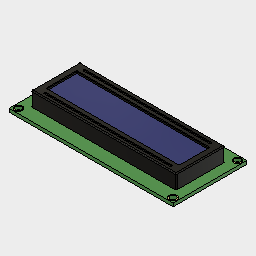
lcd_16x2 (Autodesk Fusion 360 design; units mm, degrees)
Autodesk Fusion 360 part; units mm, degrees
sketch "Sketch1" plane through (0, 0, 0) normal (0, 1, 0) x (1, 0, 0)
  line L0 (40, -18) -> (-40, -18)
  line L1 (-40, -18) -> (-40, 18)
  line L2 (-40, 18) -> (40, 18)
  line L3 (40, 18) -> (40, -18)
  line L4 (-40, -18) -> (40, 18) construction
  circle A0 centre (-37.7, 15.7) radius 1.4
  circle A1 centre (-37.7, -15.7) radius 1.4
  circle A2 centre (37.7, -15.7) radius 1.4
  circle A3 centre (37.7, 15.7) radius 1.4
  circle A4 centre (-32, 15.5) radius 0.5
  circle A5 centre (-29.46, 15.5) radius 0.5
  circle A6 centre (-26.92, 15.5) radius 0.5
  circle A7 centre (-24.38, 15.5) radius 0.5
  circle A8 centre (-21.84, 15.5) radius 0.5
  circle A9 centre (-19.3, 15.5) radius 0.5
  circle A10 centre (-16.76, 15.5) radius 0.5
  circle A11 centre (-14.22, 15.5) radius 0.5
  circle A12 centre (-11.68, 15.5) radius 0.5
  circle A13 centre (-9.14, 15.5) radius 0.5
  circle A14 centre (-6.6, 15.5) radius 0.5
  circle A15 centre (-4.06, 15.5) radius 0.5
  circle A16 centre (-1.52, 15.5) radius 0.5
  circle A17 centre (1.02, 15.5) radius 0.5
  circle A18 centre (3.56, 15.5) radius 0.5
  circle A19 centre (6.1, 15.5) radius 0.5
  dimension "d1" = 80
  dimension "d2" = 36
  dimension "d5" = 2.8
  dimension "d6" = 2.8
  dimension "d7" = 2.8
  dimension "d8" = 2.8
  dimension "d9" = 31.4
  dimension "d10" = 75.4
  dimension "d13" = 1
  dimension "d14" = 8
  dimension "d15" = 2.5
  dimension "d18" = 2.54
  dimension "d19" = 0
  measures "d1" distance of L1.end L2.end
  measures "d2" distance of L0.end L1.end
  measures "d5" diameter of A0
  measures "d6" diameter of A1
  measures "d7" diameter of A2
  measures "d8" diameter of A3
  measures "d9" distance of A0.centre A1.centre
  measures "d10" distance of A1.centre A2.centre
  measures "d13" diameter of A4
  measures "d14" distance of L1 A4.centre
  measures "d15" distance of L2 A4.centre
extrude "Extrude1" add sketch "Sketch1" along normal blind 1.6 makes body 1
sketch "Sketch2" plane through (0, 1.6, 0) normal (0, 1, 0) x (-1, 0, 0)
  circle A0 centre (-3.56, -15.5) radius 0.5
  circle A1 centre (-1.02, -15.5) radius 0.5
  circle A2 centre (1.52, -15.5) radius 0.5
  circle A3 centre (4.06, -15.5) radius 0.5
  circle A4 centre (6.6, -15.5) radius 0.5
  circle A5 centre (-6.1, -15.5) radius 0.5
  circle A6 centre (11.68, -15.5) radius 0.5
  circle A7 centre (24.38, -15.5) radius 0.5
  circle A8 centre (21.84, -15.5) radius 0.5
  circle A9 centre (19.3, -15.5) radius 0.5
  circle A10 centre (16.76, -15.5) radius 0.5
  circle A11 centre (14.22, -15.5) radius 0.5
  circle A12 centre (9.14, -15.5) radius 0.5
  circle A13 centre (26.92, -15.5) radius 0.5
  circle A14 centre (29.46, -15.5) radius 0.5
  circle A15 centre (32, -15.5) radius 0.5
  circle A16 centre (-37.7, -15.7) radius 1.4
  circle A17 centre (-37.7, 15.7) radius 1.4
  circle A18 centre (37.7, 15.7) radius 1.4
  circle A19 centre (37.7, -15.7) radius 1.4
  line L0 (-40, -18) -> (40, -18)
  line L1 (40, -18) -> (40, 18)
  line L2 (40, 18) -> (-40, 18)
  line L3 (-40, 18) -> (-40, -18)
  line L4 (-35.35, 11.9) -> (35.35, 11.9)
  line L5 (35.35, 11.9) -> (35.35, -11.9)
  line L6 (35.35, -11.9) -> (-35.35, -11.9)
  line L7 (-35.35, -11.9) -> (-35.35, 11.9)
  line L8 (-35.35, 11.9) -> (35.35, -11.9) construction
  line L9 (35.35, 11.9) -> (-35.35, -11.9) construction
  line L10 (-32.25, 7.25) -> (32.25, 7.25)
  line L11 (32.25, 7.25) -> (32.25, -7.25)
  line L12 (32.25, -7.25) -> (-32.25, -7.25)
  line L13 (-32.25, -7.25) -> (-32.25, 7.25)
  line L14 (-32.25, 7.25) -> (32.25, -7.25) construction
  line L15 (32.25, 7.25) -> (-32.25, -7.25) construction
  dimension "d20" = 70.7
  dimension "d21" = 23.8
  dimension "d22" = 64.5
  dimension "d23" = 14.5
  measures "d20" distance of L5.end L6.end
  measures "d21" distance of L4.end L5.end
  measures "d22" distance of L11.end L12.end
  measures "d23" distance of L10.end L11.end
extrude "Extrude2" add sketch "Sketch2" along normal blind 6 separate body contours L10 L11 L12 L13 makes body 2
extrude "Extrude3" add sketch "Sketch2" along normal blind 7 separate body contours L4 L5 L6 L7 makes body 3
sketch "Sketch3" plane through (0, 8.6, 0) normal (0, 1, 0) x (-1, 0, 0)
  line L0 (32.25, -7.25) -> (-32.25, -7.25)
  line L1 (-32.25, -7.25) -> (-32.25, 7.25)
  line L2 (-32.25, 7.25) -> (32.25, 7.25)
  line L3 (32.25, 7.25) -> (32.25, -7.25)
  line L4 (-35.35, -11.9) -> (35.35, -11.9)
  line L5 (35.35, -11.9) -> (35.35, 11.9)
  line L6 (35.35, 11.9) -> (-35.35, 11.9)
  line L7 (-35.35, 11.9) -> (-35.35, -11.9)
  line L8 (30.5703, -8.9649) -> (-30.5703, -8.9649)
  arc A0 (-30.5703, -8.9649) -> (-30.5703, -9.9649) centre (-30.5703, -9.4649) ccw
  line L9 (-30.5703, -9.9649) -> (30.5703, -9.9649)
  arc A1 (30.5703, -9.9649) -> (30.5703, -8.9649) centre (30.5703, -9.4649) ccw
  line L10 (30.5703, -9.4649) -> (-30.5703, -9.4649) construction
  line L11 (30.5703, 10.268) -> (-30.5703, 10.268)
  arc A2 (-30.5703, 10.268) -> (-30.5703, 9.268) centre (-30.5703, 9.768) ccw
  line L12 (-30.5703, 9.268) -> (30.5703, 9.268)
  arc A3 (30.5703, 9.268) -> (30.5703, 10.268) centre (30.5703, 9.768) ccw
  line L13 (30.5703, 9.768) -> (-30.5703, 9.768) construction
  point P0 (0, -9.4649)
  point P1 (0, 9.768)
  dimension "d28" = 1
  dimension "d29" = 1
  measures "d28" diameter of A0
  measures "d29" diameter of A2
extrude "Extrude4" cut sketch "Sketch3" against normal blind 0.5 contours L11 A2 L12 A3 bodies 2 1 3
extrude "Extrude5" cut sketch "Sketch3" against normal blind 0.5 contours L8 A0 L9 A1 bodies 2 1 3
sketch "Sketch4" plane through (0, 1.6, 0) normal (0, 1, 0) x (-1, 0, 0)
  circle A0 centre (-3.56, -15.5) radius 0.5
  circle A1 centre (-1.02, -15.5) radius 0.5
  circle A2 centre (1.52, -15.5) radius 0.5
  circle A3 centre (4.06, -15.5) radius 0.5
  circle A4 centre (6.6, -15.5) radius 0.5
  circle A5 centre (-6.1, -15.5) radius 0.5
  circle A6 centre (11.68, -15.5) radius 0.5
  circle A7 centre (24.38, -15.5) radius 0.5
  circle A8 centre (21.84, -15.5) radius 0.5
  circle A9 centre (19.3, -15.5) radius 0.5
  circle A10 centre (16.76, -15.5) radius 0.5
  circle A11 centre (14.22, -15.5) radius 0.5
  circle A12 centre (9.14, -15.5) radius 0.5
  circle A13 centre (26.92, -15.5) radius 0.5
  circle A14 centre (29.46, -15.5) radius 0.5
  circle A15 centre (32, -15.5) radius 0.5
  circle A16 centre (-37.7, -15.7) radius 1.4
  circle A17 centre (-37.7, 15.7) radius 1.4
  circle A18 centre (37.7, 15.7) radius 1.4
  circle A19 centre (37.7, -15.7) radius 1.4
  line L0 (-40, -18) -> (40, -18)
  line L1 (40, -18) -> (40, 18)
  line L2 (40, 18) -> (-40, 18)
  line L3 (-40, 18) -> (-40, -18)
  circle A20 centre (37.7, -15.7) radius 1.9
  line L4 (32.7, -15.5) -> (32.7, -18)
  line L5 (31.3, -15.5) -> (31.3, -18)
  line L6 (31.3, -18) -> (31.2918, -18)
  arc A21 (32.7, -15.5) -> (31.3, -15.5) centre (32, -15.5) ccw
  line L7 (40, -18) -> (-40, -18)
  line L8 (-40, -18) -> (-40, 18)
  line L9 (-40, 18) -> (40, 18)
  line L10 (40, 18) -> (40, -18)
  line L11 (30.16, -15.5) -> (30.16, -18)
  line L12 (28.76, -15.5) -> (28.76, -18)
  arc A22 (30.16, -15.5) -> (28.76, -15.5) centre (29.46, -15.5) ccw
  line L13 (27.62, -15.5) -> (27.62, -18)
  line L14 (26.22, -15.5) -> (26.22, -18)
  arc A23 (27.62, -15.5) -> (26.22, -15.5) centre (26.92, -15.5) ccw
  line L15 (25.08, -15.5) -> (25.08, -18)
  line L16 (23.68, -15.5) -> (23.68, -18)
  arc A24 (25.08, -15.5) -> (23.68, -15.5) centre (24.38, -15.5) ccw
  line L17 (22.54, -15.5) -> (22.54, -18)
  line L18 (21.14, -15.5) -> (21.14, -18)
  arc A25 (22.54, -15.5) -> (21.14, -15.5) centre (21.84, -15.5) ccw
  line L19 (20, -15.5) -> (20, -18)
  line L20 (18.6, -15.5) -> (18.6, -18)
  arc A26 (20, -15.5) -> (18.6, -15.5) centre (19.3, -15.5) ccw
  line L21 (17.46, -15.5) -> (17.46, -18)
  line L22 (16.06, -15.5) -> (16.06, -18)
  arc A27 (17.46, -15.5) -> (16.06, -15.5) centre (16.76, -15.5) ccw
  line L23 (14.92, -15.5) -> (14.92, -18)
  line L24 (13.52, -15.5) -> (13.52, -18)
  arc A28 (14.92, -15.5) -> (13.52, -15.5) centre (14.22, -15.5) ccw
  line L25 (12.38, -15.5) -> (12.38, -18)
  line L26 (10.98, -15.5) -> (10.98, -18)
  arc A29 (12.38, -15.5) -> (10.98, -15.5) centre (11.68, -15.5) ccw
  line L27 (9.84, -15.5) -> (9.84, -18)
  line L28 (8.44, -15.5) -> (8.44, -18)
  arc A30 (9.84, -15.5) -> (8.44, -15.5) centre (9.14, -15.5) ccw
  line L29 (7.3, -15.5) -> (7.3, -18)
  line L30 (5.9, -15.5) -> (5.9, -18)
  arc A31 (7.3, -15.5) -> (5.9, -15.5) centre (6.6, -15.5) ccw
  line L31 (4.76, -15.5) -> (4.76, -18)
  line L32 (3.36, -15.5) -> (3.36, -18)
  arc A32 (4.76, -15.5) -> (3.36, -15.5) centre (4.06, -15.5) ccw
  line L33 (2.22, -15.5) -> (2.22, -18)
  line L34 (0.82, -15.5) -> (0.82, -18)
  arc A33 (2.22, -15.5) -> (0.82, -15.5) centre (1.52, -15.5) ccw
  line L35 (-0.32, -15.5) -> (-0.32, -18)
  line L36 (-1.72, -15.5) -> (-1.72, -18)
  arc A34 (-0.32, -15.5) -> (-1.72, -15.5) centre (-1.02, -15.5) ccw
  line L37 (-2.86, -15.5) -> (-2.86, -18)
  line L38 (-4.26, -15.5) -> (-4.26, -18)
  arc A35 (-2.86, -15.5) -> (-4.26, -15.5) centre (-3.56, -15.5) ccw
  line L39 (-5.4, -15.5) -> (-5.4, -18)
  line L40 (-6.8, -15.5) -> (-6.8, -18)
  arc A36 (-5.4, -15.5) -> (-6.8, -15.5) centre (-6.1, -15.5) ccw
  circle A37 centre (-37.7, -15.7) radius 1.9
  circle A38 centre (-37.7, 15.7) radius 1.9
  circle A39 centre (37.7, 15.7) radius 1.9
  dimension "d34" = 3.8
  dimension "d37" = 1.4
  dimension "d40" = 0.0082
  dimension "d43" = -2.54
  dimension "d44" = 0
  dimension "d47" = 3.8
  dimension "d48" = 3.8
  dimension "d49" = 3.8
  measures "d34" diameter of A20
  measures "d37" diameter of A21
  measures "d40" distance of L5.end L6.end
  measures "d47" diameter of A37
  measures "d48" diameter of A38
  measures "d49" diameter of A39
extrude "Extrude6" add sketch "Sketch4" along normal blind 0.001 contours A20 bodies 2 3 1
extrude "Extrude7" add sketch "Sketch4" along normal blind 0.01 contours L0 L7 L39 L40 A36 | L0 L7 L37 L38 A35 | L0 L4 L5 A21 L7 | L0 L7 L35 L36 A34 | L0 L7 L33 L34 A33 | L0 L7 L11 L12 A22 | L0 L7 L31 L32 A32 | L0 L7 L13 L14 A23 | L0 L7 L29 L30 A31 | L0 L7 L15 L16 A24 | L0 L7 L27 L28 A30 | L0 L7 L17 L18 A25 | L0 L7 L25 L26 A29 | L0 L7 L19 L20 A26 | L0 L7 L23 L24 A28 | L0 L7 L21 L22 A27 | A37 | A38 | A39 bodies 3 2 1
fillet "Fillet1" radius 0.5 8 edges at (-35.35, 5.1, 11.9) (-35.35, 5.1, -11.9) (-35.35, 8.6, 0) (0, 8.6, 11.9) (0, 8.6, -11.9) (35.35, 5.1, 11.9) (35.35, 8.6, 0) (35.35, 5.1, -11.9) on bodies 3
fillet "Fillet2" radius 0.25 8 edges at (0, 8.6, 7.25) (-32.25, 8.6, 0) (0, 8.6, -7.25) (32.25, 8.6, 0) (32.25, 5.1, -7.25) (32.25, 5.1, 7.25) (-32.25, 5.1, -7.25) (-32.25, 5.1, 7.25) on bodies 3
